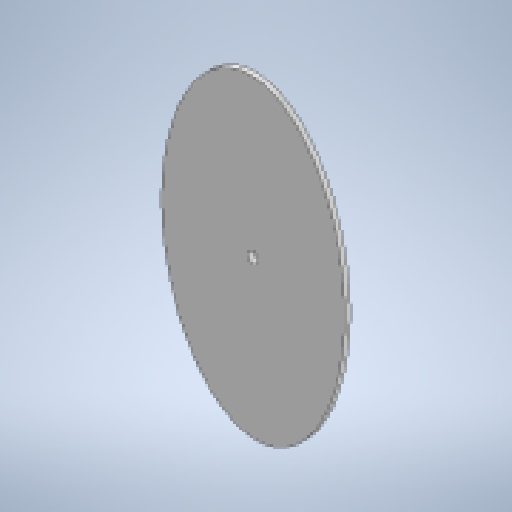
# Autodesk Inventor part: верхний эллипс туловища
Saved by Autodesk Inventor 2023.1 (Build 271208000, 208)
## iProperties
Created: 2024-11-21
Part Number: верхний эллипс туловища
Material: Типовые
Document SubType Name: Modeling
Designer: DELL
Density: 1 g/cm^3
Appearance: По умолчанию
Author: DELL
Autodesk Inventor part; units mm, degrees
ref_plane "YZ Plane" through (0, 0, 0) normal (1, 0, 0) x (0, 1, 0)
ref_plane "XZ Plane" through (0, 0, 0) normal (0, 1, 0) x (-1, 0, 0)
ref_plane "XY Plane" through (0, 0, 0) normal (0, 0, 1) x (1, 0, 0)
sketch "Эскиз1" plane through (0, 0, 0) normal (0, 0, 1) x (1, 0, 0)
  ellipse E0 centre (0, 0) end of major axis (0.8348, -119.9971) minor radius 70
  circle A0 centre (0, 0) radius 10
  line L0 (-1.5357, -9.8814) -> (-1.5357, 9.8814)
  point P0 (-2.6143, 119.9459)
  dimension "d0" = 120
  dimension "d1" = 70
  dimension "d4" = 20
  constraints: 2 coincident, 2 end point, 2 point on circle, 1 centre point, 3 other
  measures "d4" diameter of A0
extrude "Выдавливание1" add sketch "Эскиз1" against normal blind 4
sketch "Эскиз3" plane through (0, 0, 0) normal (0, 0, 1) x (1, 0, 0)
  ellipse E0 centre (0, 0) end of major axis (0.8348, -119.9971) minor radius 70 construction
  line L0 (2, 120) -> (-2, 120) construction
  line L1 (-2, 120) -> (-2, 0) construction
  line L2 (-2, -120) -> (2, -120) construction
  line L3 (2, -120) -> (2, 0) construction
  circle A0 centre (0, 0) radius 10 construction
  line L4 (2, 120) -> (-2, -120) construction
  line L5 (-2, 120) -> (2, -120) construction
  line L6 (-2, 0) -> (2, 0)
  line L7 (-2, 0) -> (-2, -120) construction
  line L8 (2, 0) -> (2, 120) construction
  line L9 (-2, -40) -> (2, -40)
  line L10 (-2, -80) -> (2, -80)
  line L11 (-2, 40) -> (2, 40)
  line L12 (-2, 80) -> (2, 80)
  line L13 (-2, -80) -> (-2, -40)
  line L14 (2, -40) -> (2, -80)
  line L15 (-2, 80) -> (-2, 40)
  line L16 (2, 40) -> (2, 80)
  point P0 (0, 40)
  point P1 (0, 80)
  point P2 (0, -40)
  point P3 (0, -80)
  dimension "d8" = 4
  dimension "d9" = 240
  dimension "d10" = 40
  dimension "d11" = 40
  dimension "d12" = 40
  dimension "d13" = 40
  constraints: 34 end point, 8 point on line, 7 midpoint, 6 parallel, 5 perpendicular, 3 collinear, 2 horizontal
  measures "d8" distance of L2.end L2.start
  measures "d9" distance of L2.start L0.end
  measures "d10" distance of point (0, 0) point (0, 40)
  measures "d11" distance of point (0, 40) point (0, 80)
  measures "d12" distance of point (0, -40) E0.centre
  measures "d13" distance of point (0, -80) point (0, -40)
extrude "Выдавливание2" cut sketch "Эскиз3" against normal blind 4
